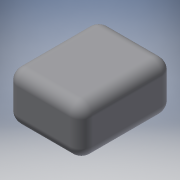
# Autodesk Inventor part: Part4
Saved by Autodesk Inventor 2018 (Build 220112000, 112)
## iProperties
Created: 2019-01-22
Part Number: Part4
Material: Generic
Document SubType Name: Modeling
Designer: petal
Density: 1 g/cm^3
Appearance: Default
Author: petal
Autodesk Inventor part; units mm, degrees
ref_plane "YZ Plane" through (0, 0, 0) normal (1, 0, 0) x (0, 1, 0)
ref_plane "XZ Plane" through (0, 0, 0) normal (0, 1, 0) x (-1, 0, 0)
ref_plane "XY Plane" through (0, 0, 0) normal (0, 0, 1) x (1, 0, 0)
sketch "Sketch1" plane through (0, 0, 0) normal (0, 1, 0) x (-1, 0, 0)
  line L0 (0, 0) -> (8.255, 0)
  line L1 (8.255, 0) -> (8.255, -10.16)
  line L2 (8.255, -10.16) -> (0, -10.16)
  line L3 (0, -10.16) -> (0, 0)
  dimension "d0" = 8.255
  dimension "d1" = 10.16
  constraints: 8 end point, 2 parallel, 1 horizontal, 1 perpendicular
  measures "d0" distance of L1.end L2.end
  measures "d1" distance of L0.end L1.end
extrude "Extrusion1" add sketch "Sketch1" along normal blind 5.334
fillet "Fillet1" radius 1.27 12 edges at (-4.1275, 5.334, 0) (0, 5.334, -5.08) (-4.1275, 5.334, -10.16) (-8.255, 5.334, -5.08) (-4.1275, 0, 0) (0, 0, -5.08) (-4.1275, 0, -10.16) (0, 2.667, -10.16) (-8.255, 2.667, -10.16) (-8.255, 2.667, 0) (-8.255, 0, -5.08) (0, 2.667, 0)
body "Solid1"
